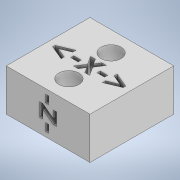
# Autodesk Inventor part: squareCalibrationBlock-25mm
Saved by Autodesk Inventor 2020.3 (Build 243373000, 373)
## iProperties
Created: 2020-06-02
Part Number: squareCalibrationBlock-25mm
Material: Generic
Document SubType Name: Modeling
Designer: robst
Density: 1 g/cm^3
Appearance: Default
Author: robst
Autodesk Inventor part; units mm, degrees
ref_plane "YZ Plane" through (0, 0, 0) normal (1, 0, 0) x (0, 1, 0)
ref_plane "XZ Plane" through (0, 0, 0) normal (0, 1, 0) x (-1, 0, 0)
ref_plane "XY Plane" through (0, 0, 0) normal (0, 0, 1) x (1, 0, 0)
sketch "Sketch1" plane through (0, 0, 0) normal (0, 1, 0) x (-1, 0, 0)
  line L0 (12.5, 12.5) -> (-12.5, 12.5)
  line L1 (-12.5, 12.5) -> (-12.5, -12.5)
  line L2 (-12.5, -12.5) -> (12.5, -12.5)
  line L3 (12.5, -12.5) -> (12.5, 12.5)
  line L4 (12.5, 12.5) -> (-12.5, -12.5) construction
  line L5 (-12.5, 12.5) -> (12.5, -12.5) construction
  point P0 (0, 0)
  dimension "d0" = 25
  dimension "d1" = 25
  constraints: 12 end point, 2 midpoint, 2 parallel, 1 horizontal, 1 perpendicular
  measures "d0" distance of L0.start L0.end
  measures "d1" distance of L1.end L0.end
extrude "Extrusion1" add sketch "Sketch1" along normal blind 12.5
sketch "Sketch2" plane through (0, 12.5, 0) normal (0, 1, 0) x (1, 0, 0)
  line L0 (-12.5, 12.5) -> (-12.5, -12.5) construction
  line L1 (-12.5, 0) -> (12.5, 0) construction
  line L2 (12.5, -12.5) -> (12.5, 12.5) construction
  line L3 (-6.1256, -2.4906) -> (-10.5058, -0.671)
  line L4 (-10.5058, -0.671) -> (-10.5058, 0.0782)
  line L5 (-10.5058, 0.0782) -> (-6.1256, 1.8978)
  line L6 (-6.1256, 1.8978) -> (-6.1256, 0.9551)
  line L7 (-6.1256, 0.9551) -> (-9.1885, -0.3005)
  line L8 (-9.1885, -0.3005) -> (-6.1256, -1.5479)
  line L9 (-6.1256, -1.5479) -> (-6.1256, -2.4906)
  line L10 (-2.7705, -0.7698) -> (-5.0306, -0.7698)
  line L11 (-5.0306, -0.7698) -> (-5.0306, 0.177)
  line L12 (-5.0306, 0.177) -> (-2.7705, 0.177)
  line L13 (-2.7705, 0.177) -> (-2.7705, -0.7698)
  line L14 (2.433, -2.54) -> (0.9592, -2.54)
  line L15 (0.9592, -2.54) -> (-0.0206, -0.9221)
  line L16 (-0.0206, -0.9221) -> (-1.0209, -2.54)
  line L17 (-1.0209, -2.54) -> (-2.433, -2.54)
  line L18 (-2.433, -2.54) -> (-0.7822, 0.0165)
  line L19 (-0.7822, 0.0165) -> (-2.3671, 2.54)
  line L20 (-2.3671, 2.54) -> (-0.8933, 2.54)
  line L21 (-0.8933, 2.54) -> (0.0247, 1.0045)
  line L22 (0.0247, 1.0045) -> (0.9674, 2.54)
  line L23 (0.9674, 2.54) -> (2.3794, 2.54)
  line L24 (2.3794, 2.54) -> (0.7863, 0.07)
  line L25 (0.7863, 0.07) -> (2.433, -2.54)
  line L26 (5.1088, -0.7698) -> (2.8488, -0.7698)
  line L27 (2.8488, -0.7698) -> (2.8488, 0.177)
  line L28 (2.8488, 0.177) -> (5.1088, 0.177)
  line L29 (5.1088, 0.177) -> (5.1088, -0.7698)
  line L30 (10.5881, -0.671) -> (6.208, -2.4906)
  line L31 (6.208, -2.4906) -> (6.208, -1.5479)
  line L32 (6.208, -1.5479) -> (9.2667, -0.2964)
  line L33 (9.2667, -0.2964) -> (6.208, 0.9551)
  line L34 (6.208, 0.9551) -> (6.208, 1.8978)
  line L35 (6.208, 1.8978) -> (10.5881, 0.0782)
  line L36 (10.5881, 0.0782) -> (10.5881, -0.671)
  point P0 (0, 0)
  constraints: 2 end point, 2 midpoint, 1 horizontal
extrude "Extrusion2" cut sketch "Sketch2" against normal blind 5.08
sketch "Sketch3" plane through (-12.5, 0, 12.5) normal (0, 0, 1) x (1, 0, 0)
  line L0 (12.4794, 12.5) -> (11.4791, 12.5) construction
  line L1 (12.5, 0) -> (12.4794, 12.5) construction
  line L2 (11.7157, 8.8011) -> (11.712, 11.0611)
  line L3 (11.712, 11.0611) -> (12.6588, 11.0627)
  line L4 (12.6588, 11.0627) -> (12.6625, 8.8026)
  line L5 (12.6625, 8.8026) -> (11.7157, 8.8011)
  line L6 (9.9531, 4.2081) -> (9.9464, 8.2342)
  line L7 (9.9464, 8.2342) -> (10.8974, 8.2357)
  line L8 (10.8974, 8.2357) -> (14.0629, 5.8986)
  line L9 (14.0629, 5.8986) -> (14.0592, 8.1174)
  line L10 (14.0592, 8.1174) -> (15.0266, 8.119)
  line L11 (15.0266, 8.119) -> (15.0328, 4.3523)
  line L12 (15.0328, 4.3523) -> (14.0654, 4.3507)
  line L13 (14.0654, 4.3507) -> (10.9164, 6.6797)
  line L14 (10.9164, 6.6797) -> (10.9205, 4.2096)
  line L15 (10.9205, 4.2096) -> (9.9531, 4.2081)
  line L16 (11.7278, 1.4404) -> (11.7241, 3.7005)
  line L17 (11.7241, 3.7005) -> (12.6709, 3.7021)
  line L18 (12.6709, 3.7021) -> (12.6746, 1.442)
  line L19 (12.6746, 1.442) -> (11.7278, 1.4404)
  constraints: 2 end point, 1 other
extrude "Extrusion3" cut sketch "Sketch3" against normal blind 5.08
sketch "Sketch11" plane through (0, 12.5, 0) normal (0, 1, 0) x (1, 0, 0)
  circle A0 centre (-0.2, 6.5) radius 3
  circle A1 centre (0.2, -6.5) radius 3
  line L0 (12.5, 12.5) -> (-12.5, 12.5) projected
  line L1 (-12.5, -12.5) -> (12.5, -12.5) projected
  point P0 (0, 0)
  dimension "d81" = 6
  dimension "d82" = 6
  dimension "d83" = 6
  constraints: 2 centre point, 1 equal radius
  measures "d81" diameter of A0
  measures "d82" distance from line of A0.centre L0
  measures "d83" distance from line of A1.centre L1
extrude "Extrusion4" cut sketch "Sketch11" against normal blind 25.4
equation "\"d46\" = 0.125 * Sketch7_Pitch"
equation "\"Sketch7_Pitch\" = 1.27"
equation "\"d48\" = 60deg"
equation "\"d67\" = 0.125 * Sketch9_Pitch"
equation "\"Sketch9_Pitch\" = 1.27"
equation "\"d69\" = 60deg"
equation "\"d99\" = 0.125 * Sketch12_Pitch"
equation "\"Sketch12_Pitch\" = 1.27"
equation "\"d101\" = 60deg"
equation "\"d120\" = 0.125 * Sketch14_Pitch"
equation "\"Sketch14_Pitch\" = 1.27"
equation "\"d122\" = 60deg"
equation "\"d143\" = 55deg"
equation "\"Sketch16_Pitch\" = 1.27"
equation "\"d161\" = 55deg"
equation "\"Sketch18_Pitch\" = 1.27"
body "Solid1"
